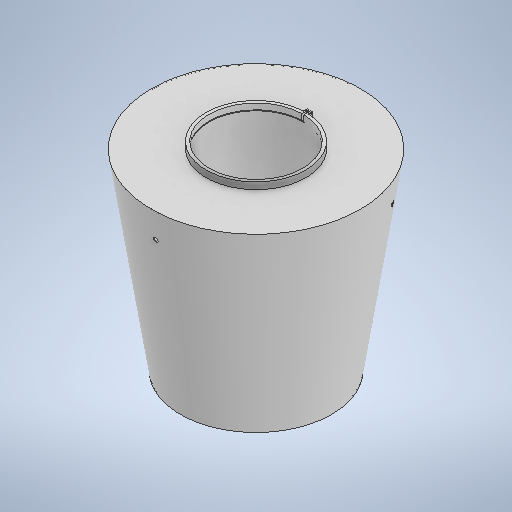
# Autodesk Inventor part: Water Sensor Bouy 4
Saved by Autodesk Inventor 2025 (Build 290162000, 162)
## iProperties
Created: 2024-06-24
Part Number: Water Sensor Bouy 4
Material: Generic
Document SubType Name: Modeling
Designer: track
Density: 1 g/cm^3
Appearance: Default
Author: track
Autodesk Inventor part; units mm, degrees
ref_plane "YZ Plane" through (0, 0, 0) normal (1, 0, 0) x (0, 1, 0)
ref_plane "XZ Plane" through (0, 0, 0) normal (0, 1, 0) x (-1, 0, 0)
sketch "Sketch2" plane through (0, 0, 0) normal (0, 0, 1) x (1, 0, 0)
  line L0 (0, 0) -> (0, 304.8)
  line L1 (61.96, 0) -> (61.96, 254)
  line L2 (61.96, 254) -> (138.16, 254)
  line L3 (138.16, 254) -> (100.06, 0)
  line L4 (100.06, 0) -> (61.96, 0)
  line L5 (136.9988, 253) -> (62.96, 253)
  line L6 (62.96, 253) -> (62.96, 1)
  line L7 (62.96, 1) -> (99.1988, 1)
  line L8 (99.1988, 1) -> (136.9988, 253)
  dimension "d2" = 304.8
  dimension "d3" = 61.96
  dimension "d4" = 76.2
  dimension "d5" = 38.1
  dimension "d7" = 254
  dimension "d8" = 0
  dimension "d9" = 1
  constraints: 18 end point, 2 parallel, 2 vertical, 1 horizontal, 3 other
  measures "d2" distance of L0.start L0.end
  measures "d3" distance between parallel lines of L0 L1
  measures "d4" distance of L1.end L2.end
  measures "d5" distance of L3.end L1.start
  measures "d7" distance of L1.start L1.end
  measures "d8" distance from line of L0.start L4
  measures "d9" distance between parallel lines of L2 L5
revolve "Revolution1" add sketch "Sketch2" angle 360 about axis through (0, 0, 0) along (0, 1, 0)
ref_plane "Work Plane1" through (0, 0, 139.7) normal (0, 0, 1) x (1, 0, 0)
sketch "Sketch3" plane through (0, 0, 139.7) normal (0, 0, 1) x (1, 0, 0)
  circle A0 centre (0, 215.9) radius 3
  line L0 (138.16, 254) -> (-138.16, 254) projected
  line L1 (0, 0) -> (0, 254)
  dimension "d12" = 6
  dimension "d13" = 38.1
  constraints: 2 end point, 1 centre point, 1 midpoint, 1 point on line
  measures "d12" diameter of A0
  measures "d13" distance from line of L0 A0.centre
extrude "Extrusion1" cut sketch "Sketch3" against normal blind 25.4
pattern_circular "Circular Pattern1" count 3 over 360 about axis through (0, 127, 0) along (0, 1, 0) of "Extrusion1"
sketch "Sketch4" plane through (0, 254, 0) normal (0, 1, 0) x (1, 0, 0)
  circle A0 centre (0, 0) radius 61.96
  circle A1 centre (0, 0) radius 61.96 projected
  circle A2 centre (0, 0) radius 65.96
  dimension "d19" = 4
  constraints: 2 centre point, 1 coincident, 1 concentric
  measures "d19" radial gap between concentric circles of A0 A2
extrude "Extrusion2" add sketch "Sketch4" along normal blind 8.89
ref_plane "Work Plane2" through (0, 254, -65.96) normal (0, 0, 1) x (1, 0, 0)
sketch "Sketch5" plane through (0, 254, -65.96) normal (0, 0, 1) x (1, 0, 0)
  line L0 (-61.96, 8.89) -> (61.96, 8.89) projected
  line L1 (138.16, 0) -> (-138.16, 0) projected
  line L2 (3.27, 8.89) -> (1.27, 8.89)
  line L3 (1.27, 8.89) -> (1.27, 0)
  line L4 (1.27, 0) -> (3.27, 0)
  line L5 (3.27, 0) -> (3.27, 8.89)
  line L6 (-1.27, 8.89) -> (-3.27, 8.89)
  line L7 (-3.27, 8.89) -> (-3.27, 0)
  line L8 (-3.27, 0) -> (-1.27, 0)
  line L9 (-1.27, 0) -> (-1.27, 8.89)
  line L10 (0, 8.89) -> (0, 0)
  point P0 (0, -254)
  point P1 (3.27, 0)
  point P2 (1.27, 8.89)
  point P3 (-1.27, 0)
  point P4 (-1.27, 8.89)
  point P5 (-3.27, 8.89)
  point P6 (-3.27, 0)
  dimension "d22" = 2
  dimension "d24" = 2.54
  constraints: 18 end point, 4 parallel, 4 point on line, 2 horizontal, 2 midpoint, 2 perpendicular, 2 other
  measures "d22" distance between parallel lines of L9 L7
  measures "d24" distance between parallel lines of L3 L9
extrude "Extrusion3" add sketch "Sketch5" along normal blind 2.54 and the other way blind 5.08 contours L0 L9 L1 L7 | L0 L5 L1 L3
sketch "Sketch7" plane through (0, 254, -65.96) normal (0, 0, 1) x (1, 0, 0)
  line L0 (1.27, 0) -> (1.27, 8.89) projected
  line L1 (-61.96, 8.89) -> (61.96, 8.89) projected
  line L2 (1.27, 0) -> (-1.27, 0)
  line L3 (-1.27, 0) -> (-1.27, 8.89)
  line L4 (-1.27, 8.89) -> (1.27, 8.89)
  line L5 (1.27, 8.89) -> (1.27, 0)
  line L6 (-1.27, 8.89) -> (-1.27, 0) projected
  point P0 (0, -254)
  dimension "d29" = 0
  constraints: 8 end point, 2 parallel, 1 horizontal, 1 perpendicular, 1 point on line
  measures "d29" distance between parallel lines of L6 L3
extrude "Extrusion4" cut sketch "Sketch7" along normal up to surface round surface about axis through (0, 127, 0) along (0, 1, 0) radius 61.96 far side no
sketch "Sketch8" plane through (3.27, 254, -65.8789) normal (1, 0, 0) x (0, 0, -1)
  line L0 (0, 8.89) -> (5.1611, 8.89) projected
  line L1 (2.6211, 8.89) -> (2.6211, 0)
  line L2 (72.2811, 0) -> (-204.0389, 0) projected
  line L3 (5.1611, 8.89) -> (5.1611, 0) projected
  circle A0 centre (2.6211, 6.985) radius 1.27
  circle A1 centre (2.6211, 3.175) radius 1.27
  point P0 (-65.8789, -254)
  dimension "d32" = 0
  dimension "d33" = 2.54
  dimension "d37" = 2.54
  dimension "d38" = 2.54
  dimension "d39" = 1.905
  dimension "d40" = 3.81
  constraints: 3 point on line, 2 centre point, 2 end point, 1 vertical
  measures "d32" distance from line of L2 L1.end
  measures "d33" distance between parallel lines of L3 L1
  measures "d37" diameter of A0
  measures "d38" diameter of A1
  measures "d39" distance from line of L0 A0.centre
  measures "d40" distance of A0.centre A1.centre
sketch "Sketch9" plane through (0, 254, -71.04) normal (0, 0, -1) x (-1, 0, 0)
  line L0 (1.27, 0) -> (1.27, 8.89) projected
  line L1 (65.96, 0) -> (65.96, 8.89) projected
  line L2 (1.27, 0) -> (65.96, 0)
  line L3 (65.96, 0) -> (65.96, 1)
  line L4 (65.96, 1) -> (1.27, 1)
  line L5 (1.27, 1) -> (1.27, 0)
  point P0 (0, -254)
  point P1 (1.27, 1)
  dimension "d34" = 1
  constraints: 8 end point, 2 parallel, 1 horizontal, 1 perpendicular, 1 point on line
  measures "d34" distance between parallel lines of L2 L4
extrude "Extrusion5" cut sketch "Sketch9" against normal blind 101.6
extrude "Extrusion6" cut sketch "Sketch8" against normal up to surface (6.54 mm away) contours A0 L1 | L1 A0 | A1 L1 | L1 A1
body "Solid1"
